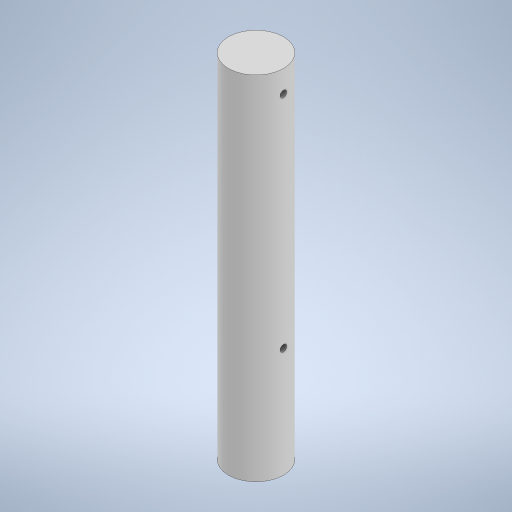
# Autodesk Inventor part: Вал
Saved by Autodesk Inventor 2023 (Build 270158000, 158)
## iProperties
Created: 2022-05-01
Part Number: Вал
Material: Типовые
Document SubType Name: Modeling
Designer: User
Density: 1 g/cm^3
Appearance: По умолчанию
Author: User
Autodesk Inventor part; units mm, degrees
ref_plane "YZ Plane" through (0, 0, 0) normal (1, 0, 0) x (0, 1, 0)
ref_plane "XZ Plane" through (0, 0, 0) normal (0, 1, 0) x (-1, 0, 0)
ref_plane "XY Plane" through (0, 0, 0) normal (0, 0, 1) x (1, 0, 0)
sketch "Эскиз1" plane through (0, 0, 0) normal (0, 1, 0) x (-1, 0, 0)
  circle A0 centre (0, 0) radius 12.5
  dimension "d0" = 25
  constraints: 1 centre point, 1 coincident
  measures "d0" diameter of A0
extrude "Выдавливание1" add sketch "Эскиз1" along normal blind 160
sketch "Эскиз2" plane through (0, 0, 0) normal (0, -1, 0) x (1, 0, 0)
  circle A0 centre (0, 0) radius 22.5
  line L0 (0, 0) -> (0, 5)
  line L1 (0, 0) -> (0, -5)
  dimension "d3" = 45
  dimension "d4" = 5
  dimension "d5" = 5
  constraints: 4 end point, 2 vertical, 1 centre point, 1 coincident
  measures "d3" diameter of A0
  measures "d4" distance of L0.start L0.end
  measures "d5" distance of L0.start L1.end
hole "Отверстие1" at (0, 0, 5) at (0, 0, -5) direction (0, 1, 0) diameter 2.459 depth 8 tip angle 118 thread size "M3x0.5" class "6H" standard "ISO Metric profile"
sketch "Эскиз4" plane through (0, 0, 0) normal (1, 0, 0) x (0, 1, 0)
  line L0 (160, -12.5) -> (160, 12.5) projected
  line L1 (160, 0) -> (150, 0)
  circle A0 centre (150, 0) radius 1.5
  line L2 (160, 0) -> (150, 0)
  line L3 (150, 0) -> (155, 0)
  circle A1 centre (145, 0) radius 1.5
  line L4 (0, 0) -> (50, 0)
  circle A2 centre (50, 0) radius 1.5
  dimension "d30" = 3
  dimension "d35" = 10
  dimension "d49" = 50
  dimension "d50" = 3
  constraints: 8 end point, 3 centre point, 3 horizontal, 2 coincident, 2 midpoint
  measures "d30" diameter of A0
  measures "d35" distance of L1.start L2.end
  measures "d49" distance of L4.start L4.end
  measures "d50" diameter of A2
extrude "Выдавливание3" cut sketch "Эскиз4" along normal mid plane 30.75 contours A0 | A2
thread "Резьба4" size "M3x0.5" class "6H" standard "ANSI Metric M Profile" full length
thread "Резьба5" size "M3x0.5" class "6H" standard "ANSI Metric M Profile" full length
